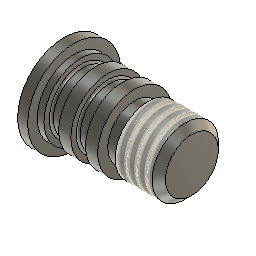
penetrator_charging (Autodesk Fusion 360 design; units mm, degrees)
Autodesk Fusion 360 part; units mm, degrees
sketch "Sketch1" plane through (0, 0, 0) normal (0, 0, 1) x (1, 0, 0)
  line L0 (0, 0) -> (65.3318, 0)
  line L1 (0, 5.5) -> (1, 5.5)
  line L2 (1, 5.5) -> (1, 4.4)
  line L3 (1, 4.4) -> (3.2, 4.4)
  line L4 (3.2, 4.4) -> (3.2, 5.5)
  line L5 (3.2, 5.5) -> (5, 5.5)
  line L6 (5, 5.5) -> (5, 4.4)
  line L7 (5, 4.4) -> (7.2, 4.4)
  line L8 (7.2, 4.4) -> (7.2, 5.5)
  line L9 (17.5, 5) -> (17.5, 0)
  line L10 (0, 5.5) -> (0, 6.9)
  line L11 (0, 6.9) -> (-1.5, 6.9)
  line L12 (-1.5, 6.9) -> (-1.5, 1.95)
  line L13 (-1.5, 1.95) -> (12.5, 1.95)
  line L14 (12.5, 1.95) -> (12.5, 0)
  line L15 (12.5, 0) -> (17.5, 0)
  line L16 (9, 5.5) -> (9, 4)
  line L17 (9, 4) -> (11, 4)
  line L18 (11, 4) -> (11, 5)
  line L19 (7.2, 5.5) -> (9, 5.5)
  line L20 (11, 5) -> (17.5, 5)
  line L21 (-1.5, 1.95) -> (-1.5, 0)
  line L22 (-1.5, 0) -> (12.5, 0)
  dimension "d1" = 1.5
  dimension "d2" = 1.4
  dimension "d3" = 1.95
  dimension "d5" = 5.5
  dimension "d9" = 1.1
  dimension "d10" = 2.2
  dimension "d11" = 1
  dimension "d12" = 1.8
  dimension "d15" = 1.8
  dimension "d16" = 2
  dimension "d25" = 5
  dimension "d26" = 19
  dimension "d32" = 14
  dimension "d33" = 6.5
  dimension "d37" = 10
  dimension "d38" = 11
  dimension "d39" = 1
  constraint coincident L0.start origin
  constraint horizontal L0
  constraint horizontal L1
  constraint perpendicular L1 L2
  constraint perpendicular L2 L3
  constraint perpendicular L1 L4
  constraint perpendicular L4 L5
  constraint perpendicular L3 L6
  constraint perpendicular L6 L7
  constraint perpendicular L5 L8
  constraint perpendicular L8 L19
  constraint perpendicular L9 L19
  constraint coincident L0 L9.end
  constraint perpendicular L1 L10
  constraint perpendicular L10 L11
  constraint perpendicular L11 L12
  constraint perpendicular L12 L13
  constraint perpendicular L13 L14
  constraint horizontal L0.start L14.end
  constraint vertical L0.start L1.start
  constraint collinear L1 L5
  constraint collinear L1 L19
  constraint collinear L3 L7
  constraint equal L3 L7
  constraint perpendicular L7 L16
  constraint perpendicular L16 L17
  constraint perpendicular L18 L19
  constraint coincident L9.end L15.end
  constraint perpendicular L0 L21
  constraint perpendicular L14 L22
  constraint horizontal L20
  measures "d1" distance of L10.end L11.end
  measures "d2" distance of L1.start L10.end
  measures "d3" distance of L0.start L13
  measures "d5" distance of L0.start L1
  measures "d9" distance of L1.end L2.end
  measures "d10" distance of L2.end L3.end
  measures "d11" distance of L0.start L2
  measures "d12" distance of L4.end L5.end
  measures "d15" distance of L8.end L16.start
  measures "d16" distance of L16.end L17.end
  measures "d25" distance of L9.end L14.end
  measures "d26" distance of L9 L12
  measures "d32" distance of L12.end L13.end
  measures "d33" distance of L9.start L18.end
  measures "d38" horizontal distance of L1.start L18.end
  measures "d39" distance of L17 L20
revolve "Revolve1" add sketch "Sketch1" angle 360 about axis through (0, 0, 0) along (1, 0, 0)
thread "Thread8" "ISO Metric profile 10.0 M10x1.5 6g" major diameter 9.85 minor diameter 8.141 pitch 1.5 angle 60 resizes the face on face at (13.1667, 4.9752, -0.4978)
chamfer "Chamfer3" distance 1 angle 45 1 edges at (17.5, -4.5917, -1.781)
hole "Hole2" at (-1.5, 0, 0) direction (1, 0, 0) diameter 4 depth 14 tip angle 118
fillet "Fillet1" radius 0.3 2 faces at (1.7333, 4.3945, -0.2193) (5.7333, 4.3945, -0.2193)
